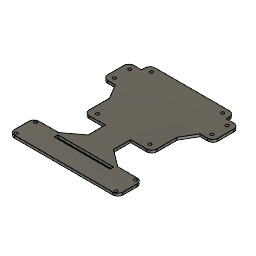
LF_Chassis (Autodesk Fusion 360 design; units mm, degrees)
part number: 2026-03-01-22-31-12-465
Autodesk Fusion 360 part; units mm, degrees
sketch "Sketch1" plane through (0, 0, 0) normal (0, 0, 1) x (1, 0, 0)
  line L0 (-44, 0) -> (44, 0)
  line L1 (-50, -6) -> (-50, -10)
  line L2 (50, -6) -> (50, -10)
  line L3 (-50, -10) -> (-59, -10)
  line L4 (50, -10) -> (59, -10)
  line L5 (-65, -16) -> (-65, -35)
  line L6 (65, -16) -> (65, -35)
  line L7 (-59, -41) -> (-50, -41)
  line L8 (59, -41) -> (50, -41)
  line L9 (40, -58) -> (50, -41)
  line L10 (-50, -41) -> (-40, -58)
  circle A0 centre (57.5, -34.525) radius 1.75
  circle A1 centre (57.5, -16.475) radius 1.75
  circle A2 centre (-57.5, -16.475) radius 1.75
  circle A3 centre (-57.5, -34.525) radius 1.75
  line L11 (-40, -58) -> (-40, -82)
  line L12 (40, -58) -> (40, -82)
  line L13 (-34, -88) -> (-15, -88)
  line L14 (34, -88) -> (15, -88)
  line L15 (-15, -88) -> (-15, -108)
  line L16 (15, -88) -> (15, -108)
  line L17 (-15, -108) -> (-15, -123) construction
  arc A4 (-44, 0) -> (-50, -6) centre (-44, -6) ccw
  arc A5 (50, -6) -> (44, 0) centre (44, -6) ccw
  arc A6 (-40, -82) -> (-34, -88) centre (-34, -82) ccw
  arc A7 (34, -88) -> (40, -82) centre (34, -82) ccw
  arc A8 (-59, -10) -> (-65, -16) centre (-59, -16) ccw
  arc A9 (-65, -35) -> (-59, -41) centre (-59, -35) ccw
  arc A10 (59, -41) -> (65, -35) centre (59, -35) ccw
  line L18 (-64, -129) -> (-64, -146)
  line L19 (64, -129) -> (64, -146)
  line L20 (-58, -152) -> (58, -152)
  line L21 (64, -126) -> (59, -126) construction
  line L22 (59, -126) -> (59, -123) construction
  circle A11 centre (59, -126) radius 1.75
  line L23 (59, -152) -> (59, -149) construction
  line L24 (59, -149) -> (64, -149) construction
  circle A12 centre (59, -149) radius 1.75
  line L25 (-64, -149) -> (-59, -149) construction
  line L26 (-59, -149) -> (-59, -152) construction
  circle A13 centre (-59, -149) radius 1.75
  line L27 (-59, -123) -> (-59, -126) construction
  line L28 (-64, -126) -> (-59, -126) construction
  circle A14 centre (-59, -126) radius 1.75
  line L29 (-58, -123) -> (-35, -123)
  line L30 (58, -123) -> (35, -123)
  line L31 (-35, -123) -> (-15, -108)
  line L32 (15, -108) -> (35, -123)
  circle A15 centre (-42, -6.5) radius 1.75
  circle A16 centre (42, -6.5) radius 1.75
  line L33 (-39.875, -81) -> (-31, -81) construction
  circle A17 centre (-31, -81) radius 1.75
  circle A18 centre (31, -81) radius 1.75
  arc A19 (65, -16) -> (59, -10) centre (59, -16) ccw
  arc A20 (-58, -123) -> (-64, -129) centre (-58, -129) ccw
  arc A21 (-64, -146) -> (-58, -152) centre (-58, -146) ccw
  arc A22 (64, -129) -> (58, -123) centre (58, -129) ccw
  arc A23 (58, -152) -> (64, -146) centre (58, -146) ccw
  line L34 (-35.1953, -126) -> (-32.7453, -126) construction
  line L35 (35, -126) -> (32.55, -126) construction
  line L36 (-32.7453, -126) -> (32.7453, -126)
  line L37 (32.7453, -126) -> (32.7453, -130)
  line L38 (32.7453, -130) -> (-32.7453, -130)
  line L39 (-32.7453, -130) -> (-32.7453, -126)
  point P0 (-50, 0)
  point P1 (50, 0)
  point P2 (-65, -10)
  point P3 (65, -10)
  point P4 (-65, -41)
  point P5 (65, -41)
  point P6 (-40, -88)
  point P7 (40, -88)
  point P8 (-64, -123)
  point P9 (64, -123)
  point P10 (-64, -152)
  point P11 (64, -152)
  dimension "d103" = 19
  dimension "d104" = 19
  dimension "d105" = 88
  dimension "d106" = 24
  dimension "d107" = 24
  dimension "d108" = 18.05
  dimension "d109" = 19
  dimension "d110" = 65.4906
  dimension "d111" = 4
  dimension "d112" = 23
  dimension "d113" = 25
  dimension "d114" = 116
  dimension "d115" = 17
  dimension "d116" = 19.7231
  constraint horizontal L0
  constraint perpendicular L0 L1
  constraint perpendicular L3 L5
  constraint perpendicular L6 L8
  constraint perpendicular L12 L14
  constraint coincident P0 L1
  constraint coincident P0 L0
  constraint coincident P1 L0
  constraint coincident P1 L2
  constraint tangent L2 A5
  constraint coincident P6 L11
  constraint coincident P6 L13
  constraint tangent L13 A6
  constraint coincident P7 L12
  constraint coincident P7 L14
  constraint tangent L12 A7
  constraint tangent L14 A7
  constraint coincident P2 L5
  constraint coincident P2 L3
  constraint coincident P4 L5
  constraint coincident P4 L7
  constraint coincident P5 L8
  constraint coincident P5 L6
  constraint tangent L8 A10
  constraint tangent L6 A10
  constraint perpendicular L19 L20
  constraint coincident L19 L21.start
  constraint coincident L21.end L22.start
  constraint coincident L19 L24.end
  constraint coincident L23.end L24.start
  constraint coincident L18 L25.start
  constraint coincident L20 L26.end
  constraint coincident L25.end L26.start
  constraint coincident L18 L28.start
  constraint coincident L27.end L28.end
  constraint coincident L33.end A17.centre
  constraint coincident P3 L4
  constraint coincident P3 L6
  constraint tangent L6 A19
  constraint coincident P8 L29
  constraint coincident P8 L18
  constraint coincident P10 L18
  constraint coincident P10 L20
  constraint tangent L20 A21
  constraint coincident P9 L30
  constraint coincident P9 L19
  constraint tangent L19 A22
  constraint coincident P11 L20
  constraint coincident P11 L19
  constraint tangent L20 A23
  constraint tangent L19 A23
  constraint horizontal L36
  constraint vertical L37
  constraint horizontal L38
  constraint vertical L39
  measures "d103" distance of L5.start L5.end
  measures "d104" distance of L6.end L6.start
  measures "d105" distance of L0.start L0.end
  measures "d106" distance of L10.end L11.end
  measures "d107" distance of L9.start L12.end
  measures "d108" distance of A0.centre A1.centre
  measures "d109" distance of L13.end L13.start
  measures "d110" distance of L34.end L36.end
  measures "d111" distance of L36.end L37.end
  measures "d112" distance of L30.end L30.start
  measures "d113" distance of L16.end L30.end
  measures "d114" distance of L20.start L20.end
  measures "d115" distance of L18.start L18.end
  measures "d116" distance of L7.end L10.end
extrude "Extrude1" add sketch "Sketch1" along normal blind 3
